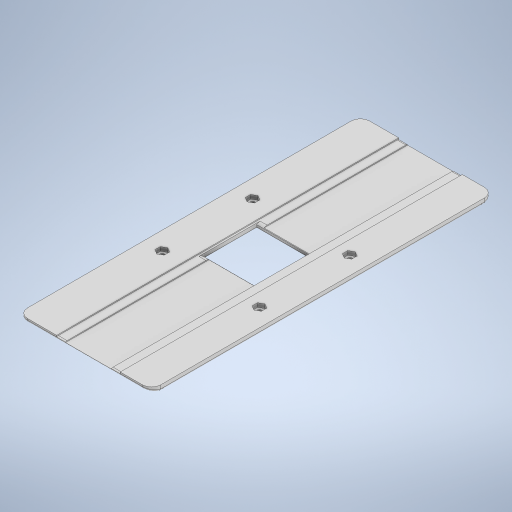
# Autodesk Inventor part: Base
Saved by Autodesk Inventor 2023 (Build 270158000, 158)
## iProperties
Created: 2026-01-10
Part Number: Base
Material: Generico
Document SubType Name: Modeling
Designer: Davide
Density: 1 g/cm^3
Appearance: Default
1_Materiale: − − −
2_Trattamento: − − −
3_Disegnato: D. Mitidieri
4_Controllato: C. Pirrottina
5_Approvato: S. Musella
Author: Davide
Autodesk Inventor part; units mm, degrees
sketch "Schizzo1" plane through (0, 0, 0) normal (0, 1, 0) x (-1, 0, 0)
  line L0 (-37, 95) -> (37, 95)
  line L1 (37, 95) -> (37, -95)
  line L2 (37, -95) -> (-37, -95)
  line L3 (-37, -95) -> (-37, 95)
  line L4 (-37, 95) -> (37, -95) construction
  line L5 (37, 95) -> (-37, -95) construction
  point P0 (0, 0)
  dimension "d0" = 74
  dimension "d1" = 190
  constraints: 12 end point, 2 midpoint, 2 parallel, 1 horizontal, 1 perpendicular
  measures "d0" distance of L0.start L0.end
  measures "d1" distance of L0.end L1.end
extrude "Estrusione1" add sketch "Schizzo1" along normal mid plane 3
sketch "Schizzo2" plane through (0, 1.5, 0) normal (0, 1, 0) x (1, 0, 0)
  line L0 (-37, -95) -> (37, -95) projected
  line L1 (19.6, 95) -> (-15.7, 95)
  line L2 (-15.7, 95) -> (-15.7, -95)
  line L3 (-15.7, -95) -> (19.6, -95)
  line L4 (19.6, -95) -> (19.6, 95)
  line L5 (-14.7, -15.075) -> (14.7, -15.075) construction
  line L6 (14.7, -15.075) -> (14.7, 15.075) construction
  line L7 (14.7, 15.075) -> (-14.7, 15.075) construction
  line L8 (-14.7, 15.075) -> (-14.7, -15.075) construction
  line L9 (37, 95) -> (-37, 95) projected
  point P0 (0, 0)
  point P1 (-14.7, 0)
  point P2 (0, -15.075)
  dimension "d4" = 35.3
  dimension "d49" = 30.15
  dimension "d50" = 29.4
  dimension "d51" = 1
  dimension "d52" = 4.9
  dimension "d57" = 19.6
  dimension "d58" = 15.7
  constraints: 16 end point, 4 parallel, 2 horizontal, 2 midpoint, 2 perpendicular, 1 collinear, 1 horizontal alignment, 1 point on line, 1 vertical alignment
  measures "d4" distance between parallel lines of L4 L2
  measures "d49" distance of L7.end L5.start
  measures "d50" distance of L6.end L7.end
  measures "d51" distance between parallel lines of L8 L2
  measures "d52" distance between parallel lines of L4 L6
  measures "d57" distance from line of point (0, 0) L4
  measures "d58" distance from line of L2 point (0, 0)
extrude "Estrusione2" cut sketch "Schizzo2" against normal blind 0.55
sketch "Schizzo3" plane through (0, 0.95, 0) normal (0, 1, 0) x (1, 0, 0)
  line L0 (-15.7, 95) -> (19.6, 95) projected
  line L1 (14.7, -95) -> (-10.8, -95)
  line L2 (-10.8, -95) -> (-10.8, 95)
  line L3 (-10.8, 95) -> (14.7, 95)
  line L4 (14.7, 95) -> (14.7, -95)
  line L5 (-15.7, -95) -> (-15.7, 95) projected
  line L6 (19.6, 95) -> (19.6, -95) projected
  line L7 (-37, -95) -> (-15.7, -95) projected
  point P0 (0, 0)
  point P1 (14.7, 95)
  dimension "d8" = 4.9
  dimension "d9" = 25.5
  dimension "d53" = 4.9
  constraints: 8 end point, 2 parallel, 1 collinear, 1 horizontal, 1 perpendicular, 1 point on line
  measures "d8" distance between parallel lines of L5 L2
  measures "d9" distance between parallel lines of L4 L2
  measures "d53" distance between parallel lines of L6 L4
extrude "Estrusione3" cut sketch "Schizzo3" against normal blind 0.5
sketch "Schizzo4" plane through (0, 1.5, 0) normal (0, 1, 0) x (1, 0, 0)
  line L0 (-14.7, -15.075) -> (14.7, -15.075)
  line L1 (14.7, -15.075) -> (14.7, 15.075)
  line L2 (14.7, 15.075) -> (-14.7, 15.075)
  line L3 (-14.7, 15.075) -> (-14.7, -15.075)
  line L4 (-15.7, -95) -> (-15.7, 95) projected
  line L5 (19.6, 95) -> (19.6, -95) projected
  point P0 (0, 0)
  point P1 (0, -15.075)
  point P2 (-14.7, 0)
  dimension "d12" = 30.15
  dimension "d13" = 29.4
  dimension "d54" = 1
  dimension "d55" = 4.9
  constraints: 8 end point, 2 midpoint, 2 parallel, 1 horizontal, 1 horizontal alignment, 1 perpendicular, 1 vertical alignment
  measures "d12" distance of L2.end L0.start
  measures "d13" distance of L0.start L0.end
  measures "d54" distance between parallel lines of L4 L3
  measures "d55" distance between parallel lines of L5 L1
extrude "Estrusione4" cut sketch "Schizzo4" against normal through all
fillet "Raccordo1" radius 5 4 edges at (37, 0, 95) (-37, 0, 95) (37, 0, -95) (-37, 0, -95)
ref_plane "Piano di lavoro1" through (-10.8, 0.95, 55.0375) normal (0, 0, 1) x (1, 0, 0)
ref_plane "Piano di lavoro2" through (-10.8, 0.95, -55.0375) normal (0, 0, 1) x (1, 0, 0)
sketch "Schizzo5" plane through (37, 1.5, 90) normal (1, 0, 0) x (0, 0, -1)
  line L0 (0, 0) -> (180, 0) projected
  line L1 (-5, -3) -> (-5, 0) projected
  line L2 (0, -3) -> (-5, -3) projected
  arc A0 (-5, -1.5) -> (1.5383, -3) centre (1.5383, 12) ccw
  line L3 (180, -3) -> (0, -3) projected
  line L4 (1.5383, -3) -> (-5, -3)
  line L5 (-5, -3.1265) -> (-5, -1.5)
  point P0 (90, -1.5)
  point P1 (1.5383, -3)
  dimension "d22" = 15
  dimension "d23" = 1.5
  constraints: 4 end point, 2 collinear, 2 point on circle, 1 centre point, 1 midpoint, 1 point on line, 1 tangent
  measures "d22" radius of A0
  measures "d23" distance of L1.end L5.end
extrude "Estrusione5" cut sketch "Schizzo5" against normal through all
mirror "Specchio1" about plane through (0, 0, 0) normal (0, 0, 1) of "Estrusione5"
sketch "Schizzo6" plane through (0, 0, 0) normal (1, 0, 0) x (0, 1, 0)
  line L0 (0.95, -95) -> (0.95, 95) projected
  line L1 (0, 95) -> (1.5, 95) projected
  arc A0 (0.95, 94.1) -> (0.65, 95) centre (-0.55, 94.1) ccw
  line L2 (0.95, -95) -> (0.95, 95) projected
  point P0 (0, 0)
  point P1 (0.95, 15.075)
  dimension "d24" = 1.5
  dimension "d25" = 0.3
  constraints: 2 point on circle, 2 point on line, 1 centre point, 1 tangent
  measures "d24" radius of A0
  measures "d25" distance from line of L0 A0.end
extrude "Estrusione6" cut sketch "Schizzo6" against normal up to surface (15.7 mm away)
ref_plane "Piano di lavoro4" through (1.95, 0.45, 95) normal (1, 0, 0) x (0, 0, -1)
mirror "Specchio2" about plane through (1.95, 0.45, 95) normal (1, 0, 0) of "Estrusione6"
mirror "Specchio8" about plane through (0, 0, 0) normal (0, 0, 1) of "Estrusione6", "Specchio2"
sketch "Schizzo7" plane through (-14.7, 1.5, 100) normal (1, 0, 0) x (0, 0, -1)
  line L0 (84.925, -1.05) -> (84.925, -3) projected
  line L1 (5.9, -0.55) -> (195, -0.55) projected
  arc A0 (84.925, -1.25) -> (82.9989, -0.55) centre (82.9989, -3.55) ccw
  line L2 (195, -0.55) -> (5.9, -0.55) projected
  line L3 (188.4617, -3) -> (11.5383, -3) projected
  point P0 (100, -1.5)
  point P1 (55, -0.55)
  point P2 (55, -3)
  point P3 (84.925, -0.55)
  point P4 (84.925, -3)
  point P5 (84.925, -0.55)
  dimension "d28" = 3
  dimension "d29" = 1.75
  constraints: 2 point on circle, 1 centre point, 1 point on line, 1 tangent, 2 other
  measures "d28" radius of A0
  measures "d29" distance from line of L3 A0.start
extrude "Estrusione7" cut sketch "Schizzo7" along normal up to surface (29.4 mm away) fills toward (84.0406, -0.6834) open curves A0
mirror "Specchio7" about plane through (0, 0, 0) normal (0, 0, 1) of "Estrusione7"
fillet "Raccordo3" radius 1 12 edges at (37, -1.4802, 89.2318) (37, -1.5, 0) (37, -1.4802, -89.2318) (35.2676, -0.5238, -93.7845) (0, 0, -95) (-35.2676, -0.5238, -93.7845) (-37, -1.4802, -89.2318) (-37, -1.5, 0) (-37, -1.4802, 89.2318) (-35.2676, -0.5238, 93.7845) (0, 0, 95) (35.2676, -0.5238, 93.7846)
sketch "Schizzo8" plane through (0, 1.5, 0) normal (0, 1, 0) x (1, 0, 0)
  line L0 (29.6, -23.5739) -> (29.6, -26.5761)
  line L1 (29.6, -26.5761) -> (27, -28.0772)
  line L2 (27, -28.0772) -> (24.4, -26.5761)
  line L3 (24.4, -26.5761) -> (24.4, -23.5739)
  line L4 (24.4, -23.5739) -> (27, -22.0728)
  line L5 (27, -22.0728) -> (29.6, -23.5739)
  line L6 (-29.6, -23.5739) -> (-27, -22.0728)
  line L7 (-27, -22.0728) -> (-24.4, -23.5739)
  line L8 (-24.4, -23.5739) -> (-24.4, -26.5761)
  line L9 (-24.4, -26.5761) -> (-27, -28.0772)
  line L10 (-27, -28.0772) -> (-29.6, -26.5761)
  line L11 (-29.6, -26.5761) -> (-29.6, -23.5739)
  line L12 (-24.4, 26.5761) -> (-24.4, 23.5739)
  line L13 (-24.4, 23.5739) -> (-27, 22.0728)
  line L14 (-27, 22.0728) -> (-29.6, 23.5739)
  line L15 (-29.6, 23.5739) -> (-29.6, 26.5761)
  line L16 (-29.6, 26.5761) -> (-27, 28.0772)
  line L17 (-27, 28.0772) -> (-24.4, 26.5761)
  line L18 (27, 28.0772) -> (29.6, 26.5761)
  line L19 (29.6, 26.5761) -> (29.6, 23.5739)
  line L20 (29.6, 23.5739) -> (27, 22.0728)
  line L21 (27, 22.0728) -> (24.4, 23.5739)
  line L22 (24.4, 23.5739) -> (24.4, 26.5761)
  line L23 (24.4, 26.5761) -> (27, 28.0772)
  point P0 (0, 0)
  point P1 (27, -25.075)
  point P2 (-27, -25.075)
  point P3 (-27, 25.075)
  point P4 (27, 25.075)
  dimension "d33" = 25.075
  dimension "d34" = 27
  dimension "d35" = 5.2
  dimension "d36" = 25.075
  dimension "d37" = 25.075
  dimension "d38" = 27
  constraints: 48 end point, 4 vertical, 3 equal length, 2 horizontal alignment, 2 vertical alignment, 52 other
  measures "d33" vertical distance of point (0, 0) point (-27, -25.075)
  measures "d34" horizontal distance of point (0, 0) point (-27, -25.075)
  measures "d35" distance between parallel lines of L8 L11
  measures "d36" vertical distance of point (0, 0) point (-27, 25.075)
  measures "d37" vertical distance of point (0, 0) point (27, 25.075)
  measures "d38" horizontal distance of point (0, 0) point (27, 25.075)
extrude "Estrusione8" cut sketch "Schizzo8" against normal blind 2.2
fillet "Raccordo4" radius 0.5 4 edges at (0, -1.5, -15.075) (0, -1.5, 15.075) (-14.7, -1.5, 0) (14.7, -1.5, 0)
sketch "Schizzo9" plane through (0, 1.5, 0) normal (0, 1, 0) x (1, 0, 0)
  line L0 (-29.6, -23.5739) -> (-27, -22.0728) projected
  circle A0 centre (-27, -25.075) radius 2.6
  line L1 (-29.6, -26.5761) -> (-29.6, -23.5739) projected
  line L2 (-27, -22.0728) -> (-24.4, -23.5739) projected
  line L3 (-24.4, -26.5761) -> (-27, -28.0772) projected
  point P0 (0, 0)
  constraints: 3 tangent, 1 centre point
sketch "Schizzo10" plane through (0, -0.7, 0) normal (0, 1, 0) x (1, 0, 0)
  line L0 (-29.6, 23.5739) -> (-29.6, 26.5761) projected
  line L1 (24.4, -26.5761) -> (24.4, -23.5739) projected
  point P0 (0, 0)
  point P1 (-27, -25.075)
  point P2 (27, -25.075)
  point P3 (-27, 25.075)
  point P4 (27, 25.075)
  point P5 (-29.6, 25.075)
  point P6 (-27, 28.0772)
  point P7 (27, -22.0728)
  point P8 (24.4, -25.075)
  constraints: 4 horizontal alignment, 4 vertical alignment, 2 midpoint
hole "Foro1" at (-27, -0.7, 25.075) at (27, -0.7, 25.075) at (-27, -0.7, -25.075) at (27, -0.7, -25.075) direction (0, -1, 0) diameter 2.8 depth 0.6
equation "\"d36\" = d33"
equation "\"d38\" = d34"
